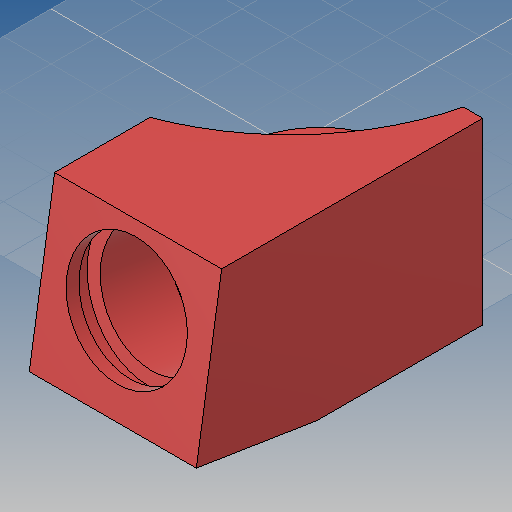
# Autodesk Inventor part: Zyklon_Stutzen
Saved by Autodesk Inventor 2019 (Build 230136000, 136)
## iProperties
Created: 2020-07-30
Part Number: Zyklon_Stutzen
Material: Generisch
Document SubType Name: Modeling
Designer: Stefan
Density: 1 g/cm^3
Appearance: Glatt - Rot
Mass: 243.682 g
Surface Area: 465.699 cm^2
Volume: 243.682 cm^3
Author: Stefan
Autodesk Inventor part; units mm, degrees
sketch "Skizze1" plane through (0, 0, 0) normal (0, 1, 0) x (-1, 0, 0)
  circle A0 centre (0, 0) radius 100
  circle A1 centre (0, 0) radius 95.1
  line L0 (-93.2, 0) -> (-47, 0) construction
  line L1 (-47, 0) -> (-47, 89.2524) construction
  line L2 (-47, 89.2524) -> (-93.2, 89.2524) construction
  line L3 (-93.2, 89.2524) -> (-93.2, 0) construction
  line L4 (-45.1, 0) -> (-95.1, 0) construction
  line L5 (-95.1, 0) -> (-95.1, 89.2524) construction
  line L6 (-95.1, 89.2524) -> (-45.1, 89.2524) construction
  line L7 (-45.1, 89.2524) -> (-45.1, 0) construction
  line L8 (-97.0145, 24.2524) -> (-105.1, 24.2524)
  line L9 (-105.1, 24.2524) -> (-105.1, 144.2524)
  line L10 (-105.1, 144.2524) -> (-35.1, 144.2524)
  line L11 (-35.1, 144.2524) -> (-35.1, 93.6375)
  line L12 (-70.1, 0) -> (-70.1, 89.2524) construction
  dimension "d0" = 200
  dimension "d1" = 4.9
  dimension "d2" = 46.2
  dimension "d3" = 50
  dimension "d6" = 55
  dimension "d39" = 10
  dimension "d40" = 120
  constraints: 26 end point, 5 perpendicular, 4 parallel, 3 horizontal, 3 midpoint, 3 point on circle, 2 coincident, 1 centre point, 1 collinear, 1 horizontal alignment, 1 vertical, 3 other
  measures "d0" diameter of A0
  measures "d2" distance of L1.end L2.end
  measures "d3" distance of L5.end L6.end
  measures "d6" distance between parallel lines of L10 L2
  measures "d39" distance between parallel lines of L7 L11
  measures "d40" distance between parallel lines of L10 L8
extrude "Extrusion1" add sketch "Skizze1" against normal blind 75 contours A0 L8 L9 L10 L11
ref_plane "Arbeitsebene1" through (95.1, 0, 89.2524) normal (0, -0.1564345, -0.9876883) x (-1, 0, 0)
sketch "Skizze2" plane through (95.1, 0, 89.2524) normal (0, -0.1564345, -0.9876883) x (-1, 0, 0)
  line L0 (25, 13.9622) -> (25, 0) construction
  circle A0 centre (25, -37.5) radius 25.1
  line L1 (0, 0) -> (50, 0) construction
  circle A1 centre (25, -37.5) radius 23.1
  point P0 (95.1, 13.9622)
  dimension "d10" = 50.2
  dimension "d11" = 37.5
  dimension "d12" = 2
  constraints: 2 centre point, 1 coincident, 1 point on line
  measures "d10" diameter of A0
  measures "d11" distance from line of A0.centre L1
  measures "d12" radial gap between concentric circles of A0 A1
extrude "Extrusion4" cut sketch "Skizze2" against normal through all contours A0 | A1
ref_plane "Arbeitsebene4" through (0, 0, 0) normal (0.7547096, 0, 0.656059) x (0, 1, 0)
sketch "Skizze4" plane through (0, 0, 0) normal (0.7547096, 0, 0.656059) x (0, 1, 0)
  line L0 (-90, 0) -> (15, 0) projected
  circle A0 centre (-37.5, 0) radius 36.5
  line L1 (0, -45.3438) -> (0, 47.6415) projected
  line L2 (0, -45.3438) -> (-75, -45.3438) projected
  line L3 (-75, 47.6415) -> (-75, -45.3438) projected
  line L4 (0, 47.6415) -> (-75, 47.6415) projected
  circle A1 centre (-37.5, 0) radius 37.5 construction
  line L5 (-70.5, -33) -> (-4.5, -33)
  line L6 (-4.5, -33) -> (-4.5, 33)
  line L7 (-4.5, 33) -> (-70.5, 33)
  line L8 (-70.5, 33) -> (-70.5, -33)
  line L9 (-70.5, -33) -> (-4.5, 33) construction
  line L10 (-4.5, -33) -> (-70.5, 33) construction
  circle A2 centre (-4.5, -33) radius 3
  circle A3 centre (-4.5, 33) radius 3
  circle A4 centre (-70.5, 33) radius 3
  circle A5 centre (-70.5, -33) radius 3
  point P0 (0, 0)
  dimension "d27" = 73
  dimension "d35" = 6
  dimension "d36" = 66
  constraints: 12 end point, 6 centre point, 5 coincident, 3 equal radius, 3 midpoint, 2 parallel, 2 perpendicular, 2 tangent, 1 horizontal
  measures "d27" diameter of A0
  measures "d35" diameter of A2
  measures "d36" distance of L5.end L6.end
extrude "Extrusion8" add sketch "Skizze4" along normal up to surface contours A0 L8 L0 | L0 L8 A0 | L8 A0 L7 L6 L0 | L0 L6 A0 L5 L8 | L6 A0 L0 | L0 A0 L6 | A0 L7 | L5 A0
extrude "Extrusion9" cut sketch "Skizze1" against normal through all contours A1
extrude "Extrusion10" cut sketch "Skizze2" along normal through all contours A1
extrude "Extrusion11" cut sketch "Skizze4" along normal blind 106 contours A4 L7 L8 | L8 L7 A4 | A5 L5 L8 | L8 L5 A5 | A2 L5 L6 | L6 L5 A2 | A3 L7 L6 | L6 L7 A3
sketch "Skizze6" plane through (35.1, 0, 93.6375) normal (-1, 0, 0) x (0, 0, 1)
  line L0 (0, 0) -> (50.6148, 0) projected
  line L1 (50.6148, 0) -> (40.0057, 0)
  line L2 (50.6148, -75) -> (0, -75) projected
  line L3 (50.6148, 0) -> (50.6148, -66.9834)
  line L4 (50.6148, -66.9834) -> (40.0057, 0)
  line L5 (0, -75) -> (50.6148, -66.9834)
  line L6 (50.6148, -66.9834) -> (50.6148, -75)
  line L7 (0, -75) -> (50.6148, -75)
  point P0 (-93.6375, 0)
  dimension "d44" = 9
  dimension "d45" = 9
  constraints: 12 end point, 1 collinear, 1 perpendicular, 1 point on line, 1 vertical
  measures "d44" angle of L3 L4
  measures "d45" angle of L2 L5
extrude "Extrusion12" cut sketch "Skizze6" against normal through all
ref_plane "Arbeitsebene6" through (35.1, -1.5643, 123.7664) normal (0, 0.1564345, 0.9876883) x (1, 0, 0)
sketch "Skizze7" plane through (35.1, -1.5643, 123.7664) normal (0, 0.1564345, 0.9876883) x (1, 0, 0)
  line L0 (70, -67.8184) -> (0, -67.8184) projected
  line L1 (0, -67.8184) -> (0, 1.5838) projected
  line L2 (0, 1.5838) -> (70, 1.5838) projected
  line L3 (70, 1.5838) -> (70, -67.8184) projected
  circle A0 centre (35, -30.5557) radius 25.1 projected
  circle A1 centre (35, -30.5557) radius 30.5
  point P0 (-35.1, 20.9064)
  dimension "d47" = 61
  constraints: 1 centre point, 1 coincident
  measures "d47" diameter of A1
extrude "Extrusion13" cut sketch "Skizze7" along normal mid plane 9 contours A1
equation "\"d0\" = kg_diameter"
equation "\"d1\" = kg_thickness"
equation "\"d2\" = ht_diameter - 2 * ht_thickness"
equation "\"d3\" = ht_diameter"
equation "\"d10\" = ht_diameter + 2 * gap_fit"
equation "\"d12\" = ht_thickness + gap_fit"
equation "\"d27\" = bore_diameter"
equation "\"d45\" = d44"
equation "\"kg_diameter\" = 200"
equation "\"kg_thickness\" = 4.9"
equation "\"ht_diameter\" = 50"
equation "\"ht_thickness\" = 1.9"
equation "\"case_thickness\" = 18"
equation "\"gap_air\" = 1"
equation "\"gap_slide\" = 0.2"
equation "\"gap_fit\" = 0.1"
equation "\"bore_diameter\" = 73"
equation "\"tape_width\" = 15"
equation "\"tape_thickness\" = 3"
equation "\"mdf_thickness\" = 6"
equation "\"inner_thickness\" = 15"
equation "\"inner_depth\" = 255"
